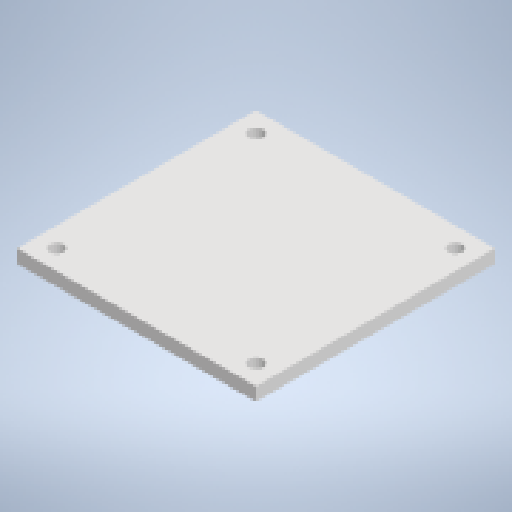
# Autodesk Inventor part: 飞控外壳
Saved by Autodesk Inventor 2025.2 (Build 292293000, 293)
## iProperties
Created: 2026-04-16
Part Number: 飞控外壳
Material: 常规
Document SubType Name: Modeling
Designer: BO‘S_SLAVE
Density: 1 g/cm^3
Appearance: 默认
Author: BO‘S_SLAVE
Autodesk Inventor part; units mm, degrees
ref_plane "YZ Plane" through (0, 0, 0) normal (1, 0, 0) x (0, 1, 0)
ref_plane "XZ Plane" through (0, 0, 0) normal (0, 1, 0) x (-1, 0, 0)
ref_plane "XY Plane" through (0, 0, 0) normal (0, 0, 1) x (1, 0, 0)
sketch "草图1" plane through (0, 0, 0) normal (0, 1, 0) x (-1, 0, 0)
  line L0 (0, 0) -> (-36, 0)
  line L1 (-36, 0) -> (-36, -36)
  line L2 (-36, -36) -> (0, -36)
  line L3 (0, -36) -> (0, 0)
  circle A0 centre (-3, -3) radius 1.05
  line L4 (0, -18) -> (-36, -18)
  line L5 (-18, 0) -> (-18, -36)
  circle A1 centre (-3, -33) radius 1.05
  circle A2 centre (-33, -3) radius 1.05
  circle A3 centre (-33, -33) radius 1.05
  dimension "d0" = 36
  dimension "d1" = 36
  dimension "d2" = 2.1
  dimension "d6" = 3
  dimension "d7" = 3
  constraints: 12 end point, 4 centre point, 4 midpoint, 3 symmetric about line, 2 parallel, 1 horizontal, 1 perpendicular, 3 other
  measures "d0" distance between parallel lines of L1 L3
  measures "d1" distance between parallel lines of L2 L0
  measures "d2" diameter of A0
  measures "d6" distance from line of L3 A0.centre
  measures "d7" distance from line of L0 A0.centre
extrude "拉伸1" add sketch "草图1" along normal blind 2
